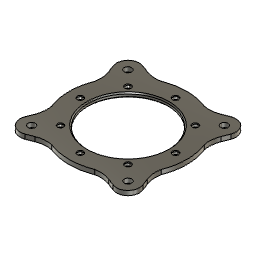
Motor_Base_Plate_Top v1 (Autodesk Fusion 360 design; units mm, degrees)
Autodesk Fusion 360 part; units mm, degrees
sketch "Sketch1" plane through (0, 0, 0) normal (0, 0, 1) x (1, 0, 0)
  circle A0 centre (0, 0) radius 52.5
  line L0 (-52.5, 52.5) -> (52.5, 52.5)
  line L1 (52.5, 52.5) -> (52.5, -52.5)
  line L2 (52.5, -52.5) -> (-52.5, -52.5)
  line L3 (-52.5, -52.5) -> (-52.5, 52.5)
  line L4 (-52.5, 52.5) -> (52.5, -52.5) construction
  line L5 (52.5, 52.5) -> (-52.5, -52.5) construction
  circle A1 centre (0, 0) radius 42.5 construction
  circle A2 centre (0, 0) radius 35.75
  circle A3 centre (0, 42.5) radius 1.5
  circle A4 centre (-30.052, 30.052) radius 1.5
  circle A5 centre (-42.5, 0) radius 1.5
  circle A6 centre (-30.052, -30.052) radius 1.5
  circle A7 centre (0, -42.5) radius 1.5
  circle A8 centre (30.052, -30.052) radius 1.5
  circle A9 centre (42.5, 0) radius 1.5
  circle A10 centre (30.052, 30.052) radius 1.5
  dimension "d1" = 105
  dimension "d2" = 105
  dimension "d3" = 105
  dimension "d4" = 85
  dimension "d5" = 71.5
  dimension "d7" = 3
  dimension "d9" = 360
  constraint coincident A0.centre A1.centre
  constraint horizontal L0
  constraint perpendicular L0 L1
  constraint parallel L0 L2
  constraint parallel L1 L3
  constraint coincident L4 A0.centre
  constraint coincident L5 A0.centre
  constraint concentric A0 A1
  constraint coincident A1 A3.centre
  measures "d1" diameter of A0
  measures "d2" distance of L1.end L2.end
  measures "d3" distance of L0.end L1.end
  measures "d4" diameter of A1
  measures "d5" diameter of A2
  measures "d7" diameter of A3
extrude "Mounting_face_Extrude1" add sketch "Sketch1" along normal blind 4 contours A0
chamfer "Inner_hole_Chamfer" distance 1 angle 45 2 edges at (-33.3307, 12.9278, 4) (-33.3307, 12.9278, 0)
sketch "Sketch3" plane through (0, 0, 4) normal (0, 0, 1) x (-1, 0, 0)
  circle A0 centre (0, 0) radius 36.75
  circle A1 centre (0, 0) radius 52.5
  line L0 (0, 0) -> (37.1231, -37.1231) construction
  line L1 (0, 0) -> (52.5, 0) construction
  line L2 (54.8008, -19.4454) -> (19.4454, -54.8008) construction
  line L3 (37.1231, -37.1231) -> (49.3231, -37.1231) construction
  line L4 (37.1231, -37.1231) -> (28.4964, -45.7498)
  line L5 (28.4964, -45.7498) -> (45.7498, -28.4964)
  line L6 (45.7498, 28.4964) -> (28.4964, 45.7498)
  line L7 (19.4454, 54.8008) -> (54.8008, 19.4454) construction
  line L8 (-28.4964, 45.7498) -> (-45.7498, 28.4964)
  line L9 (-54.8008, 19.4454) -> (-19.4454, 54.8008) construction
  line L10 (-45.7498, -28.4964) -> (-28.4964, -45.7498)
  line L11 (-19.4454, -54.8008) -> (-54.8008, -19.4454) construction
  circle A2 centre (30.052, -30.052) radius 1.5
  circle A3 centre (42.5, 0) radius 1.5
  circle A4 centre (0, -42.5) radius 1.5
  circle A5 centre (30.052, 30.052) radius 1.5
  circle A6 centre (-42.5, 0) radius 1.5
  circle A7 centre (-30.052, -30.052) radius 1.5
  circle A8 centre (0, 42.5) radius 1.5
  circle A9 centre (-30.052, 30.052) radius 1.5
  circle A10 centre (42.5, 0) radius 2.75
  circle A11 centre (30.052, 30.052) radius 2.75
  circle A12 centre (0, 42.5) radius 2.75
  circle A13 centre (-30.052, 30.052) radius 2.75
  circle A14 centre (-42.5, 0) radius 2.75
  circle A15 centre (-30.052, -30.052) radius 2.75
  circle A16 centre (0, -42.5) radius 2.75
  circle A17 centre (30.052, -30.052) radius 2.75
  point P0 (28.4964, -45.7498)
  point P1 (45.7498, -28.4964)
  point P2 (45.7498, 28.4964)
  point P3 (28.4964, 45.7498)
  point P4 (-28.4964, 45.7498)
  point P5 (-45.7498, 28.4964)
  point P6 (-45.7498, -28.4964)
  point P7 (-28.4964, -45.7498)
  dimension "d24" = 45
  dimension "d26" = 25
  dimension "d31" = 12.2
  dimension "d71" = 360
  dimension "d115" = 5.5
  dimension "d117" = 360
  constraint horizontal L1
  constraint coincident A0.centre A1.centre
  constraint coincident A1 L0.end
  constraint symmetric L0 L2.start L2.end
  constraint horizontal L3
  constraint symmetric L3.start L0 L4.start
  constraint symmetric L0 P1 P0
  constraint coincident P0 L4.end
  constraint coincident P1 L5.end
  constraint concentric A3 A10
  measures "d24" angle of L0 L1
  measures "d26" distance of L0.end L2.start
  measures "d31" distance of L0.end P1
  measures "d115" diameter of A10
sketch "Sketch5" plane through (0, 0, 4) normal (0, 0, 1) x (1, 0, 0)
  line L0 (-45.7498, 28.4964) -> (-63.0032, 45.7498) construction
  line L1 (0, 0) -> (-37.1231, 37.1231)
  line L2 (-28.4964, 45.7498) -> (-45.7617, 62.9913) construction
  line L3 (-42.0139, 59.2438) -> (-59.2438, 42.0139) construction
  arc A0 (-42.0139, 59.2438) -> (-59.2438, 42.0139) centre (-50.6288, 50.6288) ccw construction
  arc A1 (-45.7617, 62.9913) -> (-63.0032, 45.7498) centre (-54.3825, 54.3706) ccw construction
  line L4 (-45.7617, 62.9913) -> (-42.0139, 59.2438) construction
  line L5 (-63.0032, 45.7498) -> (-59.2438, 42.0139) construction
  line L6 (-54.3765, 37.1231) -> (-50.0632, 32.8098) construction
  circle A2 centre (0, 0) radius 52.5 construction
  line L7 (-50.0632, 32.8098) -> (-48.8708, 19.1807) construction
  line L8 (-50.0632, 32.8098) -> (-41.1648, 32.8098) construction
  line L9 (-32.8098, 50.0632) -> (-19.1807, 48.8708) construction
  arc A3 (-48.8708, 19.1807) -> (-50.0632, 32.8098) centre (-73.2053, 23.9184) ccw
  arc A4 (-32.8098, 50.0632) -> (-19.1807, 48.8708) centre (-23.9184, 73.2053) ccw
  line L10 (-37.1231, 37.1231) -> (-42.9921, 42.9921) construction
  line L11 (-37.1231, 37.1231) -> (-18.8231, 37.1231) construction
  circle A5 centre (-42.9921, 42.9921) radius 3.3
  line L12 (-45.7498, 28.4964) -> (-44.7336, 27.4802) construction
  line L13 (-45.7498, 28.4964) -> (-44.3126, 28.4964) construction
  line L14 (-28.4964, 45.7498) -> (-27.4802, 44.7336) construction
  arc A6 (-27.4802, 44.7336) -> (-48.8708, 19.1807) centre (0, 0) ccw construction
  arc A7 (-19.1807, 48.8708) -> (-48.8708, 19.1807) centre (0, 0) ccw
  line L15 (-52.5, 0) -> (-71.6, 0) construction
  line L16 (-50.0632, 32.8098) -> (-52.5813, 39.2323)
  line L17 (-32.8098, 50.0632) -> (-39.2323, 52.5813)
  arc A8 (-39.2323, 52.5813) -> (-52.5813, 39.2323) centre (-42.9921, 42.9921) ccw
  line L18 (-50.0632, -32.8098) -> (-52.5813, -39.2323)
  arc A9 (-50.0632, -32.8098) -> (-48.8708, -19.1807) centre (-73.2053, -23.9184) ccw
  arc A10 (-44.7336, -27.4802) -> (-19.1807, -48.8708) centre (0, 0) ccw construction
  arc A11 (-48.8708, -19.1807) -> (-19.1807, -48.8708) centre (0, 0) ccw
  arc A12 (-19.1807, -48.8708) -> (-32.8098, -50.0632) centre (-23.9184, -73.2053) ccw
  line L19 (-32.8098, -50.0632) -> (-39.2323, -52.5813)
  arc A13 (-52.5813, -39.2323) -> (-39.2323, -52.5813) centre (-42.9921, -42.9921) ccw
  circle A14 centre (-42.9921, -42.9921) radius 3.3
  line L20 (-37.1231, -37.1231) -> (-42.9921, -42.9921) construction
  line L21 (32.8098, -50.0632) -> (39.2323, -52.5813)
  arc A15 (32.8098, -50.0632) -> (19.1807, -48.8708) centre (23.9184, -73.2053) ccw
  arc A16 (27.4802, -44.7336) -> (48.8708, -19.1807) centre (0, 0) ccw construction
  arc A17 (19.1807, -48.8708) -> (48.8708, -19.1807) centre (0, 0) ccw
  arc A18 (48.8708, -19.1807) -> (50.0632, -32.8098) centre (73.2053, -23.9184) ccw
  line L22 (50.0632, -32.8098) -> (52.5813, -39.2323)
  arc A19 (39.2323, -52.5813) -> (52.5813, -39.2323) centre (42.9921, -42.9921) ccw
  circle A20 centre (42.9921, -42.9921) radius 3.3
  line L23 (37.1231, -37.1231) -> (42.9921, -42.9921) construction
  line L24 (50.0632, 32.8098) -> (52.5813, 39.2323)
  arc A21 (50.0632, 32.8098) -> (48.8708, 19.1807) centre (73.2053, 23.9184) ccw
  arc A22 (44.7336, 27.4802) -> (19.1807, 48.8708) centre (0, 0) ccw construction
  arc A23 (48.8708, 19.1807) -> (19.1807, 48.8708) centre (0, 0) ccw
  arc A24 (19.1807, 48.8708) -> (32.8098, 50.0632) centre (23.9184, 73.2053) ccw
  line L25 (32.8098, 50.0632) -> (39.2323, 52.5813)
  arc A25 (52.5813, 39.2323) -> (39.2323, 52.5813) centre (42.9921, 42.9921) ccw
  circle A26 centre (42.9921, 42.9921) radius 3.3
  line L26 (37.1231, 37.1231) -> (42.9921, 42.9921) construction
  line L27 (71.1, 0) -> (50.5, 0) construction
  point P0 (-45.7498, 28.4964)
  point P1 (-59.2438, 59.2438)
  point P2 (-50.0632, 32.8098)
  point P3 (-54.3765, 37.1231)
  point P4 (-85.5492, 19.4221)
  point P5 (-32.8098, 50.0632)
  point P6 (-37.1231, 54.3765)
  point P7 (-32.8098, 50.0632)
  point P8 (-50.6288, 50.6288)
  point P9 (-52.5, 0)
  point P10 (-50.2753, 50.2753)
  point P11 (-37.1231, 37.1231)
  point P12 (-50.2753, -50.2753)
  point P13 (-48.8708, -19.1807)
  point P14 (-50.0632, -32.8098)
  point P15 (-32.8098, -50.0632)
  point P16 (50.2753, -50.2753)
  point P17 (19.1807, -48.8708)
  point P18 (32.8098, -50.0632)
  point P19 (50.0632, -32.8098)
  point P20 (50.2753, 50.2753)
  point P21 (48.8708, 19.1807)
  point P22 (50.0632, 32.8098)
  point P23 (32.8098, 50.0632)
  dimension "d36" = 6.1
  dimension "d37" = 85
  dimension "d38" = 135
  dimension "d39" = 8.3
  dimension "d40" = 6.6
  dimension "d41" = 45
  dimension "d65" = 19.1
  dimension "d94" = 18.6
  dimension "d96" = 360
  dimension "d97" = 20.6
  constraint coincident P0 L0.start
  constraint symmetric P0 L1 L2.start
  constraint symmetric L3.end L1 L3.start
  constraint midpoint L3 A0.centre
  constraint midpoint A0 P1
  constraint midpoint L0 P3
  constraint coincident P2 L6.end
  constraint horizontal L8
  constraint coincident A2 L7.end
  constraint coincident P3 L6.start
  constraint symmetric L1 P2 P7
  constraint symmetric L1 L7.end L9.end
  constraint symmetric L1 P3 P6
  constraint coincident P2 A3
  constraint symmetric L1 A3 A4
  constraint horizontal L11
  constraint coincident P11 L1.end
  constraint coincident P7 P5
  constraint coincident L10.end A5.centre
  constraint horizontal L13
  constraint coincident A2 L12.end
  constraint symmetric L10 P0 L2.start
  constraint symmetric L10 L12.end L14.end
  constraint coincident P11 A6
  constraint coincident P11 A7
  constraint coincident A0.centre P8
  constraint coincident P9 L15.start
  constraint concentric A5 A8
  constraint tangent L16 A8
  constraint symmetric L10 P2 P7
  constraint symmetric L10 L16.end L17.end
  constraint midpoint A8 P10
  constraint horizontal L27
  measures "d36" distance of P3 P2
  measures "d37" angle of L7 L8
  measures "d38" angle of L10 L11
  measures "d39" distance of P11 L10.end
  measures "d40" diameter of A5
  measures "d41" angle of L12 L13
  measures "d65" distance of P9 L15.end
  measures "d94" distance of P10 P11
  measures "d97" distance of L27.start L27.end
extrude "Extrude6" add sketch "Sketch5" against normal blind 4
chamfer "Chamfer4" distance 0.5 angle 45 8 edges at (28.6535, 30.5945, 4) (-1.3985, 43.0424, 4) (41.1015, 0.5424, 4) (28.6535, -29.5096, 4) (-1.3985, -41.9576, 4) (-31.4505, -29.5096, 4) (-43.8985, 0.5424, 4) (-31.4505, 30.5945, 4)
extrude "Extrude9" cut sketch "Sketch3" against normal blind 1 contours A10 | A11 | A12 | A13 | A14 | A15 | A16 | A17
chamfer "Chamfer5" distance 1.25 angle 45 8 edges at (-1.3985, 41.9576, 3) (-31.4505, 29.5096, 3) (-31.4505, -30.5945, 3) (-43.8985, -0.5424, 3) (-1.3985, -43.0424, 3) (28.6535, -30.5945, 3) (41.1015, -0.5424, 3) (28.6535, 29.5096, 3)
equation "d31 = ( 36.6 / 3 ) * 1 mm"
equation "d36 = 12.200 mm / 2"
equation "d39 = 5 mm + 3.3 mm"
equation "d97 = 10.300 mm * 2"
